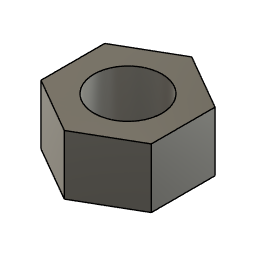
rubber feet v1 (Autodesk Fusion 360 archive; units mm, degrees)
design "M8 nut"
Autodesk Fusion 360 part; units mm, degrees
sketch "Sketch1" plane through (0, 0, 0) normal (0, 1, 0) x (1, 0, 0)
  line L0 (-6.5, -3.7528) -> (0, -7.5056)
  line L1 (0, -7.5056) -> (6.5, -3.7528)
  line L2 (6.5, -3.7528) -> (6.5, 3.7528)
  line L3 (6.5, 3.7528) -> (0, 7.5056)
  line L4 (0, 7.5056) -> (-6.5, 3.7528)
  line L5 (-6.5, 3.7528) -> (-6.5, -3.7528)
  circle A0 centre (0, 0) radius 4
  dimension "d1" = 13
  dimension "d2" = 8
  constraint coincident A0.centre origin
  measures "d1" distance of L2 L5
  measures "d2" diameter of A0
extrude "Extrude1" add sketch "Sketch1" along normal blind 7
named bodies: "M8 nut"
